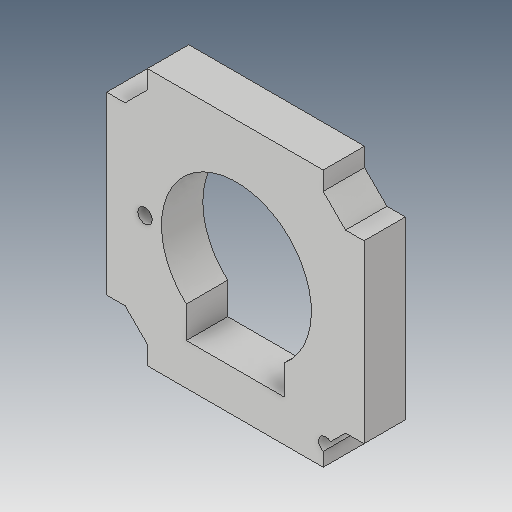
# Autodesk Inventor part: 20_Cube_Insert_RaspiCam_v3
Saved by Autodesk Inventor 2019.4 (Build 234330000, 330)
## iProperties
Created: 2019-07-01
Part Number: 20_Cube_Insert_RaspiCam_v3
Material: Generic
Document SubType Name: Modeling
Designer: diederichbenedict
Density: 1 g/cm^3
Appearance: Default
Author: diederichbenedict
Autodesk Inventor part; units mm, degrees
ref_plane "YZ Plane" through (0, 0, 0) normal (1, 0, 0) x (0, 1, 0)
ref_plane "XZ Plane" through (0, 0, 0) normal (0, 1, 0) x (-1, 0, 0)
ref_plane "Work Plane1" through (0, 0, 10) normal (0, 0, 1) x (1, 0, 0)
sketch "Sketch1" plane through (0, 0, 10) normal (0, 0, 1) x (1, 0, 0)
  line L0 (-4.0299, -0.3538) -> (-2.2322, 1.4439) construction
  arc A0 (-1.4439, 2.2322) -> (-2.2322, 1.4439) centre (-0.9299, 0.9299) ccw construction
  line L1 (-1.4439, 2.2322) -> (0.3538, 4.0299) construction
  line L2 (-37.8299, 42.2137) -> (-37.8299, 45.8299) construction
  line L3 (-37.8299, 45.8299) -> (-4.0299, 45.8299) construction
  line L4 (-4.0299, 45.8299) -> (-4.0299, 42.2137) construction
  line L5 (-4.0299, 4.0299) -> (0.3538, 4.0299) projected
  circle A1 centre (-20.9299, 20.9299) radius 17.5 construction
  line L6 (-20.9299, 58.9723) -> (17.1124, 20.9299) construction
  line L7 (17.1124, 20.9299) -> (-20.9299, -17.1124) construction
  line L8 (-20.9299, -17.1124) -> (-58.9723, 20.9299) construction
  line L9 (-58.9723, 20.9299) -> (-20.9299, 58.9723) construction
  line L10 (-20.9299, 58.9723) -> (-20.9299, -17.1124) construction
  line L11 (17.1124, 20.9299) -> (-58.9723, 20.9299) construction
  line L12 (-20.9299, 58.9723) -> (32.8701, 58.9723) construction
  line L13 (-43.2198, 43.4299) -> (1.7802, 43.4299) construction
  line L14 (1.7802, 43.4299) -> (1.7802, -1.5701) construction
  line L15 (1.7802, -1.5701) -> (-43.2198, -1.5701) construction
  line L16 (-43.2198, -1.5701) -> (-43.2198, 43.4299) construction
  line L17 (-43.2198, 5.1774) -> (-43.2198, 36.6824)
  line L18 (-43.2198, 36.6824) -> (-36.4723, 43.4299)
  line L19 (-36.4723, 43.4299) -> (-5.3876, 43.4299)
  line L20 (-5.3876, 43.4299) -> (1.7802, 36.2621)
  line L21 (1.7802, 36.2621) -> (1.7802, 5.5977)
  line L22 (1.7802, 5.5977) -> (-5.3876, -1.5701)
  line L23 (-5.3876, -1.5701) -> (-36.4723, -1.5701)
  line L24 (-36.4723, -1.5701) -> (-43.2198, 5.1774)
  line L25 (-4.0299, 42.2137) -> (-37.8299, 42.2137) projected
  line L26 (-4.0299, -0.3538) -> (-4.0299, 4.0299) projected
  circle A2 centre (-20.7198, 20.9299) radius 7.0417 construction
  arc A3 (-7.3745, 3.5) -> (-34.4854, 3.5) centre (-20.9299, 0) ccw construction
  arc A4 (-11.4668, 9.7661) -> (-30.4087, 10.1422) centre (-20.7198, 20.9299) ccw
  line L27 (-30.5806, 10.1422) -> (-30.4087, 10.1422)
  line L28 (-30.4087, 10.1422) -> (-30.4087, 1.6029)
  line L29 (-30.4087, 1.6029) -> (-11.4668, 1.6029)
  line L30 (-11.4668, 1.6029) -> (-11.4668, 9.7661)
  line L31 (-43.2198, 43.4299) -> (-10.4667, 10.6769) construction
  line L32 (-8.5595, 8.5517) -> (1.7802, -1.5701) construction
  line L33 (1.7802, 43.4299) -> (-25.699, 15.9507) construction
  line L34 (-30.9728, 10.6769) -> (-43.2198, -1.5701) construction
  point P0 (-37.8299, 4.0299)
  dimension "d18" = 53.8
  dimension "d19" = 45
  dimension "d20" = 53.8
  dimension "d21" = 45
  dimension "d22" = 45
  dimension "d68" = 29
  constraints: 54 end point, 20 point on line, 6 parallel, 5 point on circle, 4 perpendicular, 3 horizontal, 2 midpoint, 1 centre point, 1 coincident, 1 equal length, 5 other
  measures "d18" distance of L6.start L6.end
  measures "d19" angle of L6 L12
  measures "d20" distance of L6.end L7.end
  measures "d21" distance of L14.end L15.end
  measures "d22" distance of L13.end L14.end
  measures "d68" diameter of A4
extrude "Extrusion1" add sketch "Sketch1" along normal blind 8
sketch "Sketch3" plane through (0, 0, 10) normal (0, 0, -1) x (-1, 0, 0)
  line L0 (37.8299, -0.4701) -> (37.8299, 4.0299) construction
  line L1 (4.0299, 4.0299) -> (4.0299, -0.4701) construction
  line L2 (37.8299, -0.4701) -> (37.8299, 1.1886) construction
  line L3 (4.0299, -3.9701) -> (4.0299, -0.3538) construction
  line L4 (45.8299, 4.0299) -> (42.2137, 4.0299) construction
  line L5 (-0.3538, 4.0299) -> (-3.9701, 4.0299) construction
  line L6 (-3.9701, 37.8299) -> (-0.3538, 37.8299) construction
  line L7 (4.0299, 42.2137) -> (4.0299, 45.8299) construction
  line L8 (37.8299, 45.8299) -> (37.8299, 42.2137) construction
  line L9 (42.2137, 37.8299) -> (45.8299, 37.8299) construction
  line L10 (37.8299, 37.7299) -> (45.8299, 37.7299)
  line L11 (45.8299, 37.7299) -> (45.8299, 4.1299)
  line L12 (45.8299, 4.1299) -> (37.8299, 4.1299)
  line L13 (37.8299, 4.1299) -> (37.8299, 37.7299)
  line L14 (37.7299, 4.0299) -> (4.1299, 4.0299)
  line L15 (4.1299, 4.0299) -> (4.1299, -3.9701)
  line L16 (4.1299, -3.9701) -> (37.7299, -3.9701)
  line L17 (37.7299, -3.9701) -> (37.7299, 4.0299)
  line L18 (4.0299, 4.1299) -> (-3.9701, 4.1299)
  line L19 (-3.9701, 4.1299) -> (-3.9701, 37.7299)
  line L20 (-3.9701, 37.7299) -> (4.0299, 37.7299)
  line L21 (4.0299, 37.7299) -> (4.0299, 4.1299)
  line L22 (4.1299, 37.8299) -> (37.7299, 37.8299)
  line L23 (37.7299, 37.8299) -> (37.7299, 45.8299)
  line L24 (37.7299, 45.8299) -> (4.1299, 45.8299)
  line L25 (4.1299, 45.8299) -> (4.1299, 37.8299)
  point P0 (0, 0)
  dimension "d23" = 0.1
  dimension "d24" = 0.1
  dimension "d25" = 0.1
  dimension "d26" = 0.1
  dimension "d27" = 0.1
  constraints: 32 end point, 8 parallel, 4 horizontal, 4 perpendicular, 3 point on line
  measures "d23" distance between parallel lines of L8 L23
  measures "d24" distance between parallel lines of L7 L25
  measures "d25" distance between parallel lines of L6 L20
  measures "d26" distance between parallel lines of L5 L18
  measures "d27" distance between parallel lines of L1 L15
extrude "Extrusion3" add sketch "Sketch3" against normal up to surface (8 mm away)
sketch "Skizze12" plane through (0, 0, 10) normal (0, 0, -1) x (-1, 0, 0)
  line L0 (-0.3124, 4.1299) -> (4.1299, -0.3124) projected
  line L1 (4.1299, -0.3124) -> (4.1299, -3.9701) projected
  line L2 (4.1299, -3.9701) -> (37.7299, -3.9701) construction
  line L3 (37.7299, -3.9701) -> (37.7299, -0.3124) projected
  line L4 (37.7299, -0.3124) -> (42.1723, 4.1299) projected
  line L5 (45.8299, 4.1299) -> (42.1723, 4.1299) projected
  line L6 (45.8299, 37.7299) -> (45.8299, 4.1299) construction
  line L7 (42.1723, 37.7299) -> (45.8299, 37.7299) projected
  line L8 (42.1723, 37.7299) -> (37.7299, 42.1723) projected
  line L9 (37.7299, 42.1723) -> (37.7299, 45.8299) projected
  line L10 (37.7299, 45.8299) -> (4.1299, 45.8299) construction
  line L11 (4.1299, 45.8299) -> (4.1299, 42.1723) projected
  line L12 (4.1299, 42.1723) -> (-0.3124, 37.7299) projected
  line L13 (-3.9701, 37.7299) -> (-0.3124, 37.7299) projected
  line L14 (-3.9701, 4.1299) -> (-3.9701, 37.7299) construction
  line L15 (-0.3124, 4.1299) -> (-3.9701, 4.1299) projected
  line L16 (37.9299, -4.1701) -> (3.9299, -4.1701) construction
  line L17 (3.9299, -4.1701) -> (3.9299, -0.3953)
  line L18 (3.9299, -0.3953) -> (-0.3953, 3.9299)
  line L19 (-0.3953, 3.9299) -> (-4.1701, 3.9299)
  line L20 (-4.1701, 3.9299) -> (-4.1701, 37.9299) construction
  line L21 (-4.1701, 37.9299) -> (-0.3953, 37.9299)
  line L22 (-0.3953, 37.9299) -> (3.9299, 42.2551)
  line L23 (3.9299, 42.2551) -> (3.9299, 46.0299)
  line L24 (3.9299, 46.0299) -> (37.9299, 46.0299) construction
  line L25 (37.9299, 46.0299) -> (37.9299, 42.2551)
  line L26 (37.9299, 42.2551) -> (42.2551, 37.9299)
  line L27 (42.2551, 37.9299) -> (46.0299, 37.9299)
  line L28 (46.0299, 37.9299) -> (46.0299, 3.9299) construction
  line L29 (46.0299, 3.9299) -> (42.2551, 3.9299)
  line L30 (42.2551, 3.9299) -> (37.9299, -0.3953)
  line L31 (37.9299, -0.3953) -> (37.9299, -4.1701)
  line L32 (-3.9701, 37.7299) -> (-3.9701, 37.9299)
  line L33 (37.7299, 45.8299) -> (4.1299, 45.8299) projected
  line L34 (4.1299, 45.8299) -> (3.9299, 45.8299)
  line L35 (37.7299, 45.8299) -> (37.9299, 45.8299)
  line L36 (45.8299, 37.7299) -> (45.8299, 37.9299)
  line L37 (45.8299, 4.1299) -> (45.8299, 3.9299)
  line L38 (37.7299, -3.9701) -> (37.9299, -3.9701)
  line L39 (4.1299, -3.9701) -> (3.9299, -3.9701)
  line L40 (-3.9701, 4.1299) -> (-3.9701, 3.9299)
  point P0 (0, 0)
  dimension "d65" = 0.2
  constraints: 48 end point, 13 point on line, 2 perpendicular, 1 vertical, 15 other
  measures "d65" distance between parallel lines of L2 L16
extrude "IM_offset" add sketch "Skizze12" against normal up to surface (8 mm away)
sketch "Sketch14" plane through (0, 0, 10) normal (0, 0, -1) x (-1, 0, 0)
  arc A0 (5.5299, 0) -> (1.3299, 0) centre (3.4299, 0) ccw projected
  line L0 (37.8999, 16.97) -> (37.8999, -16.97) projected
  circle A1 centre (38.3947, 20.9299) radius 1.4
  circle A2 centre (3.4299, 0) radius 1.4
  point P0 (0, 0)
  dimension "d69" = 2.8
  dimension "d70" = 2.8
  constraints: 2 centre point, 1 coincident
  measures "d69" diameter of A1
  measures "d70" diameter of A2
extrude "Extrusion12" cut sketch "Sketch14" against normal blind 10
body "Solid1"
